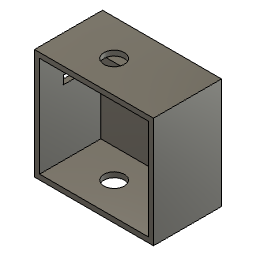
base_pata (Autodesk Fusion 360 design; units mm, degrees)
Autodesk Fusion 360 part; units mm, degrees
sketch "Sketch1" plane through (0, 0, 0) normal (0, 0, 1) x (1, 0, 0)
  line L0 (0, 0) -> (70, 0)
  line L1 (70, 0) -> (70, 65)
  line L2 (70, 65) -> (0, 65)
  line L3 (0, 65) -> (0, 0)
  dimension "d1_1" = 70
  dimension "d2_1" = 65
  constraint horizontal L0
  constraint vertical L1
  constraint horizontal L2
  constraint vertical L3
  constraint coincident L0.start L3.end
  measures "d1_1" distance of L0.start L0.end
  measures "d2_1" distance of L0.start L2.end
extrude "Extrude1" add sketch "Sketch1" along normal blind 40
shell "Shell1" thickness 3 removed faces 1 at (23.3333, 43.3333, 40)
sketch "Sketch3" plane through (0, 0, 3) normal (0, 0, 1) x (-1, 0, 0)
  line L0 (-3, -3) -> (-67, -3)
  line L1 (-67, -3) -> (-67, -62)
  line L2 (-67, -62) -> (-3, -62)
  line L3 (-3, -62) -> (-3, -3)
  line L4 (-10, -52.9161) -> (-60, -52.9161)
  line L5 (-60, -52.9161) -> (-60, -10)
  line L6 (-60, -10) -> (-10, -10)
  line L7 (-10, -10) -> (-10, -52.9161)
  dimension "d13" = 7
  dimension "d14" = 7
  dimension "d15" = 50
  constraint horizontal L4
  constraint vertical L5
  constraint horizontal L6
  constraint vertical L7
  measures "d13" distance of L0 L6
  measures "d14" distance of L3 L7
  measures "d15" distance of L5.end L6.end
extrude "Extrude2" add sketch "Sketch3" along normal blind 8 contours L4 L5 L6 L7
sketch "Sketch4" plane through (0, 0, 0) normal (0, -1, 0) x (1, 0, 0)
  line L0 (0, 0) -> (70, 0)
  line L1 (70, 0) -> (70, 40)
  line L2 (70, 40) -> (0, 40)
  line L3 (0, 40) -> (0, 0)
  circle A0 centre (28, 21.15) radius 6
  dimension "d8" = 21.15
  dimension "d9" = 28
  dimension "d10" = 12
  measures "d8" vertical distance of L0.start A0.centre
  measures "d9" horizontal distance of L0.start A0.centre
  measures "d10" diameter of A0
extrude "Extrude3" cut sketch "Sketch4" against normal blind 65 contours A0
sketch "Sketch5" plane through (0, 0, 0) normal (-1, 0, 0) x (0, 0, 1)
  line L0 (0, 65) -> (0, 0)
  line L1 (0, 0) -> (40, 0)
  line L2 (40, 0) -> (40, 65)
  line L3 (40, 65) -> (0, 65)
  line L4 (16, 46.5) -> (26, 46.5)
  line L5 (26, 46.5) -> (26, 41.5)
  line L6 (26, 41.5) -> (16, 41.5)
  line L7 (16, 41.5) -> (16, 46.5)
  dimension "d16" = 16
  dimension "d17" = 18.5
  dimension "d18" = 10
  dimension "d19" = 5
  constraint horizontal L4
  constraint vertical L5
  constraint horizontal L6
  constraint vertical L7
  measures "d16" horizontal distance of L0.start L4.start
  measures "d17" vertical distance of L0.start L4.start
  measures "d18" distance of L4.start L4.end
  measures "d19" distance of L4.start L6.end
extrude "Extrude4" cut sketch "Sketch5" against normal blind 3 contours L4 L5 L6 L7
